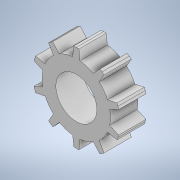
# Autodesk Inventor part: Part13
Saved by Autodesk Inventor 2021 (Build 250183000, 183)
## iProperties
Created: 2022-12-09
Part Number: Part13
Material: Generic
Document SubType Name: Modeling
Designer: user
Density: 1 g/cm^3
Appearance: Default
Author: user
Autodesk Inventor part; units mm, degrees
ref_plane "YZ Plane" through (0, 0, 0) normal (1, 0, 0) x (0, 1, 0)
ref_plane "XZ Plane" through (0, 0, 0) normal (0, 1, 0) x (-1, 0, 0)
ref_plane "XY Plane" through (0, 0, 0) normal (0, 0, 1) x (1, 0, 0)
sketch "Sketch1" plane through (0, 0, 0) normal (0, 0, 1) x (1, 0, 0)
  circle A0 centre (0, 0) radius 15
  arc A1 (-2.6749, 24.8565) -> (-12.4462, 21.6816) centre (0, 0) ccw
  arc A2 (-16.7743, 18.5371) -> (-22.8133, 10.2251) centre (0, 0) ccw
  arc A3 (12.4462, 21.6816) -> (2.6749, 24.8565) centre (0, 0) ccw
  arc A4 (22.8133, 10.2251) -> (16.7743, 18.5371) centre (0, 0) ccw
  arc A5 (24.4665, -5.1371) -> (24.4665, 5.1371) centre (0, 0) ccw
  arc A6 (16.7743, -18.5371) -> (22.8133, -10.2251) centre (0, 0) ccw
  arc A7 (2.6749, -24.8565) -> (12.4462, -21.6816) centre (0, 0) ccw
  arc A8 (-12.4462, -21.6816) -> (-2.6749, -24.8565) centre (0, 0) ccw
  arc A9 (-22.8133, -10.2251) -> (-16.7743, -18.5371) centre (0, 0) ccw
  arc A10 (-24.4665, 5.1371) -> (-24.4665, -5.1371) centre (0, 0) ccw
  line L0 (-16.7743, 18.5371) -> (-20.306, 24.7319)
  line L1 (-20.306, 24.7319) -> (-18.8091, 25.8885)
  line L2 (-18.8091, 25.8885) -> (-17.2465, 26.9547)
  line L3 (-17.2465, 26.9547) -> (-12.4462, 21.6816)
  line L4 (-24.4665, 5.1371) -> (-30.9649, 8.0729)
  line L5 (-30.9649, 8.0729) -> (-30.4338, 9.8885)
  line L6 (-30.4338, 9.8885) -> (-29.7963, 11.6696)
  line L7 (-29.7963, 11.6696) -> (-22.8133, 10.2251)
  line L8 (-22.8133, -10.2251) -> (-29.7963, -11.6696)
  line L9 (-29.7963, -11.6696) -> (-30.4338, -9.8885)
  line L10 (-30.4338, -9.8885) -> (-30.9649, -8.0729)
  line L11 (-30.9649, -8.0729) -> (-24.4665, -5.1371)
  line L12 (-12.4462, -21.6816) -> (-17.2465, -26.9547)
  line L13 (-17.2465, -26.9547) -> (-18.8091, -25.8885)
  line L14 (-18.8091, -25.8885) -> (-20.306, -24.7319)
  line L15 (-20.306, -24.7319) -> (-16.7743, -18.5371)
  line L16 (2.6749, -24.8565) -> (1.8909, -31.9441)
  line L17 (1.8909, -31.9441) -> (0, -32)
  line L18 (0, -32) -> (-1.8909, -31.9441)
  line L19 (-1.8909, -31.9441) -> (-2.6749, -24.8565)
  line L20 (16.7743, -18.5371) -> (20.306, -24.7319)
  line L21 (20.306, -24.7319) -> (18.8091, -25.8885)
  line L22 (18.8091, -25.8885) -> (17.2465, -26.9547)
  line L23 (17.2465, -26.9547) -> (12.4462, -21.6816)
  line L24 (24.4665, -5.1371) -> (30.9649, -8.0729)
  line L25 (30.9649, -8.0729) -> (30.4338, -9.8885)
  line L26 (30.4338, -9.8885) -> (29.7963, -11.6696)
  line L27 (29.7963, -11.6696) -> (22.8133, -10.2251)
  line L28 (22.8133, 10.2251) -> (29.7963, 11.6696)
  line L29 (29.7963, 11.6696) -> (30.4338, 9.8885)
  line L30 (30.4338, 9.8885) -> (30.9649, 8.0729)
  line L31 (30.9649, 8.0729) -> (24.4665, 5.1371)
  line L32 (12.4462, 21.6816) -> (17.2465, 26.9547)
  line L33 (17.2465, 26.9547) -> (18.8091, 25.8885)
  line L34 (18.8091, 25.8885) -> (20.306, 24.7319)
  line L35 (20.306, 24.7319) -> (16.7743, 18.5371)
  line L36 (-2.6749, 24.8565) -> (-1.8909, 31.9441)
  line L37 (-1.8909, 31.9441) -> (0, 32)
  line L38 (0, 32) -> (1.8909, 31.9441)
  line L39 (1.8909, 31.9441) -> (2.6749, 24.8565)
  point P0 (-2.6749, 24.8565)
  point P1 (-12.4462, 21.6816)
  point P2 (-16.7743, 18.5371)
  point P3 (-22.8133, 10.2251)
  point P4 (-24.4665, -5.1371)
  point P5 (-22.8133, -10.2251)
  point P6 (-16.7743, -18.5371)
  point P7 (-12.4462, -21.6816)
  point P8 (-2.6749, -24.8565)
  point P9 (12.4462, -21.6816)
  point P10 (16.7743, -18.5371)
  point P11 (22.8133, -10.2251)
  point P12 (24.4665, 5.1371)
  point P13 (22.8133, 10.2251)
  point P14 (16.7743, 18.5371)
  point P15 (12.4462, 21.6816)
  point P16 (2.6749, 24.8565)
  constraints: 80 end point, 20 point on circle, 11 centre point
extrude "Extrusion1" add sketch "Sketch1" along normal blind 20
body "Solid1"
